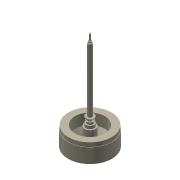
# Autodesk Inventor part: plunger
Saved by Autodesk Inventor 2022 Beta2 (Build 260130000, 130) ContinuousBuild 0
## iProperties
Shininess: 64.0
Length Units: 11272
Angle Units: 11279
Time Units: 11290
Mass Units: 11286
Length Display Precision: 3
Angle Display Precision: 2
Compacted: True
Part Number: plunger
Document SubType Name: Modeling
Created: 2003-04-07
Designer: demo
Density: 1 g/cm^3
Material: Generic
Appearance: Light Beige
Density: 0.0
Volumn: 0.0
Area: 0.0
PropertySet Name: Model Information
Control State: 0
Master: False
Checked Out: False
Author: demo
Autodesk Inventor part; units mm, degrees
ref_plane "YZ Plane" through (0, 0, 0) normal (1, 0, 0) x (0, 1, 0)
sketch "Sketch1" plane through (0, 0, 0) normal (0, 0, 1) x (1, 0, 0)
  line L0 (152.6339, -58.2676) -> (152.6339, -92.0496) projected
  line L1 (151.7318, -58.2676) -> (152.6339, -58.2676) projected
  line L2 (151.7318, -48.9712) -> (151.7318, -58.2676) projected
  line L3 (136.4664, -48.9712) -> (136.4664, -74.3712) projected
  line L4 (136.4664, -74.3712) -> (120.4816, -90.3561) projected
  line L5 (120.4816, -90.3561) -> (101.6, -90.3561) projected
  line L6 (101.6, -95.4786) -> (101.6, -90.3561) projected
  line L7 (116.0071, -95.4786) -> (101.6, -95.4786) projected
  line L8 (116.0071, -92.0496) -> (116.0071, -95.4786) projected
  line L9 (152.6339, -92.0496) -> (116.0071, -92.0496) projected
  line L10 (151.7318, -48.9712) -> (136.4664, -48.9712)
  constraints: 2 end point, 1 parallel
revolve "Revolution1" add sketch "Sketch1" angle 360 about axis through (101.6, -95.4786, 0) along (0, 1, 0)
sketch "Sketch2" plane through (101.6, -90.3561, 0) normal (0, 1, 0) x (1, 0, 0)
  circle A0 centre (0, 0) radius 14.4071 projected
extrude "Extrusion1" add sketch "Sketch2" along normal blind 7.62
sketch "Sketch3" plane through (101.6, -82.7361, 0) normal (0, 1, 0) x (1, 0, 0)
  circle A0 centre (0, 0) radius 14.4071 projected
  circle A1 centre (0, 0) radius 12.7
  dimension "d3" = 25.4
  constraints: 1 centre point, 1 coincident, 1 concentric
  measures "d3" diameter of A1
extrude "Extrusion2" add sketch "Sketch3" along normal blind 31.75 contours A1
sketch "Sketch4" plane through (101.6, -50.9861, 0) normal (0, 1, 0) x (1, 0, 0)
  circle A0 centre (0, 0) radius 12.7 projected
  circle A1 centre (0, 0) radius 9.525
  dimension "d6" = 19.05
  constraints: 1 centre point, 1 coincident, 1 concentric
  measures "d6" diameter of A1
extrude "Extrusion3" add sketch "Sketch4" along normal blind 6.604 contours A1
sketch "Sketch6" plane through (101.6, -44.3821, 0) normal (0, 1, 0) x (1, 0, 0)
  circle A0 centre (0, 0) radius 9.525 projected
  circle A1 centre (0, 0) radius 6.858
  dimension "d12" = 13.716
  constraints: 1 centre point, 1 coincident, 1 concentric
  measures "d12" diameter of A1
extrude "Extrusion5" add sketch "Sketch6" along normal blind 4.8768 contours A1
sketch "Sketch7" plane through (101.6, -39.5053, 0) normal (0, 1, 0) x (1, 0, 0)
  circle A0 centre (0, 0) radius 6.858 projected
  circle A1 centre (0, 0) radius 7.9629
  dimension "d15" = 15.9258
  constraints: 1 centre point, 1 coincident, 1 concentric
  measures "d15" diameter of A1
extrude "Extrusion6" add sketch "Sketch7" along normal blind 0.6985 contours A0 | A1
sketch "Sketch8" plane through (101.6, -38.8068, 0) normal (0, 1, 0) x (1, 0, 0)
  circle A0 centre (0, 0) radius 7.9629 projected
  circle A1 centre (0, 0) radius 5.1562
  dimension "d18" = 10.3124
  constraints: 1 centre point, 1 coincident, 1 concentric
  measures "d18" diameter of A1
extrude "Extrusion7" add sketch "Sketch8" along normal blind 7.8232 draft 30 contours A1
sketch "Sketch9" plane through (101.6, -30.9836, 0) normal (0, 1, 0) x (1, 0, 0)
  circle A0 centre (0, 0) radius 9.6729 projected
  circle A1 centre (0, 0) radius 4.9784
  dimension "d21" = 9.9568
  constraints: 1 centre point, 1 coincident, 1 concentric
  measures "d21" diameter of A1
extrude "Extrusion8" add sketch "Sketch9" along normal blind 146.2532 contours A1
sketch "Sketch10" plane through (101.6, 115.2696, 0) normal (0, 1, 0) x (1, 0, 0)
  circle A0 centre (0, 0) radius 4.9784 projected
  circle A1 centre (0, 0) radius 3.2639
  dimension "d24" = 6.5278
  constraints: 1 centre point, 1 coincident, 1 concentric
  measures "d24" diameter of A1
extrude "Extrusion9" add sketch "Sketch10" along normal blind 0.1925 contours A1
sketch "Sketch11" plane through (101.6, 115.4622, 0) normal (0, 1, 0) x (1, 0, 0)
  circle A0 centre (0, 0) radius 3.2639 projected
  circle A1 centre (0, 0) radius 4.3688
  dimension "d27" = 8.7376
  constraints: 1 centre point, 1 coincident, 1 concentric
  measures "d27" diameter of A1
extrude "Extrusion10" add sketch "Sketch11" along normal blind 1.8796 contours A0 | A1
chamfer "Chamfer1" distance 0.1981 distance2 0.1981 1 edges at (97.2312, 117.3418, 0) measured on face at (105.9122, 116.7152, 0.7008)
chamfer "Chamfer2" distance 0.1981 distance2 0.1981 1 edges at (97.2312, 115.4622, 0) measured on face at (105.5266, 115.4622, 0.6089)
sketch "Sketch12" plane through (101.6, 117.3418, 0) normal (0, 1, 0) x (1, 0, 0)
  circle A0 centre (0, 0) radius 4.1707 projected
  circle A1 centre (0, 0) radius 3.2385
  dimension "d34" = 6.477
  constraints: 1 centre point, 1 coincident, 1 concentric
  measures "d34" diameter of A1
extrude "Extrusion11" add sketch "Sketch12" along normal blind 0.2794 draft 45 contours A1
sketch "Sketch13" plane through (101.6, 117.6212, 0) normal (0, 1, 0) x (1, 0, 0)
  circle A0 centre (0, 0) radius 3.5179 projected
extrude "Extrusion12" add sketch "Sketch13" along normal blind 0.2261
sketch "Sketch14" plane through (101.6, 117.8472, 0) normal (0, 1, 0) x (1, 0, 0)
  circle A0 centre (0, 0) radius 3.5179 projected
extrude "Extrusion13" add sketch "Sketch14" along normal blind 2.0828
ref_plane "Work Plane1" through (101.6, 117.6212, 0) normal (0, 0, -1) x (0, 1, 0)
sketch "Sketch15" plane through (101.6, 117.6212, 0) normal (0, 0, -1) x (0, 1, 0)
  line L0 (0, 3.5179) -> (2.3089, 3.5179) projected
  line L1 (1.1544, 3.5179) -> (1.1544, 4.8361)
  circle A0 centre (1.1544, 4.8361) radius 1.7414
  constraints: 2 end point, 1 centre point, 1 midpoint, 1 perpendicular
ref_plane "Work Plane2" through (105.1179, 118.7756, 0) normal (0, 1, 0) x (1, 0, 0)
sketch "Sketch16" plane through (105.1179, 118.7756, 0) normal (0, 1, 0) x (1, 0, 0)
  circle A0 centre (-3.5179, 0) radius 3.5179 projected
sweep "Sweep1" cut profiles "Sketch15" path "Sketch16"
sketch "Sketch17" plane through (101.6, 119.93, 0) normal (0, 1, 0) x (1, 0, 0)
  circle A0 centre (0, 0) radius 3.5179 projected
extrude "Extrusion14" add sketch "Sketch17" along normal blind 1.143
chamfer "Chamfer3" distance 0.2286 distance2 0.2286 1 edges at (98.0821, 121.073, 0) measured on face at (105.0723, 120.3, 0.5643)
sketch "Sketch18" plane through (101.6, 121.073, 0) normal (0, 1, 0) x (1, 0, 0)
  circle A0 centre (0, 0) radius 3.2893 projected
  circle A1 centre (0, 0) radius 1.8372
  dimension "d48" = 3.6744
  constraints: 1 centre point, 1 coincident, 1 concentric
  measures "d48" diameter of A1
extrude "Extrusion15" add sketch "Sketch18" along normal blind 1.4478 contours A1
chamfer "Chamfer4" distance 0.4318 distance2 0.2286 1 edges at (99.7628, 122.5208, 0) measured on face at (101.0889, 122.0382, -1.7647)
sketch "Sketch19" plane through (101.6, 122.5208, 0) normal (0, 1, 0) x (1, 0, 0)
  circle A0 centre (0, 0) radius 1.6086 projected
  circle A1 centre (0, 0) radius 1.5875
  dimension "d53" = 3.175
  constraints: 1 centre point, 1 coincident, 1 concentric
  measures "d53" diameter of A1
extrude "Extrusion16" add sketch "Sketch19" along normal blind 11.3284 contours A1
sketch "Sketch20" plane through (101.6, 133.8492, 0) normal (0, 1, 0) x (1, 0, 0)
  circle A0 centre (0, 0) radius 1.5875 projected
extrude "Extrusion17" add sketch "Sketch20" along normal blind 4.2164 draft -20
body "Solid1"
